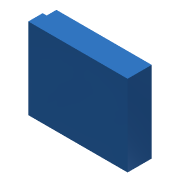
# Autodesk Inventor part: body_encoder
Saved by Autodesk Inventor 2014 (Build 180170000, 170)
## iProperties
Created: 2015-11-19
Part Number: body_encoder
Material: Generic
Document SubType Name: Modeling
Designer: Tom
Density: 1 g/cm^3
Appearance: Default
Author: Tom
Autodesk Inventor part; units mm, degrees
ref_plane "YZ Plane" through (0, 0, 0) normal (1, 0, 0) x (0, 1, 0)
ref_plane "XZ Plane" through (0, 0, 0) normal (0, 1, 0) x (-1, 0, 0)
sketch "Sketch1" plane through (0, 0, 0) normal (0, 0, 1) x (1, 0, 0)
  line L0 (0, 0) -> (12.6492, 0)
  line L1 (12.6492, 0) -> (12.6492, 11.176)
  line L2 (12.6492, 11.176) -> (0, 11.176)
  line L3 (0, 11.176) -> (0, 0)
  dimension "d0" = 12.6492
  dimension "d1" = 11.176
  constraints: 8 end point, 2 parallel, 1 horizontal, 1 perpendicular
  measures "d0" distance of L2.end L1.end
  measures "d1" distance of L1.end L0.end
extrude "Extrusion1" add sketch "Sketch1" along normal blind 3.9624
sketch "Sketch2" plane through (0, 0, 0) normal (-1, 0, 0) x (0, 0, 1)
  line L0 (0, 0) -> (3.9624, 0) projected
  line L1 (3.9624, 11.176) -> (2.0574, 11.176)
  line L2 (2.0574, 11.176) -> (2.0574, 0)
  line L3 (2.0574, 0) -> (3.9624, 0)
  line L4 (3.9624, 0) -> (3.9624, 11.176)
  dimension "d4" = 1.905
  constraints: 8 end point, 2 parallel, 1 horizontal, 1 perpendicular, 1 point on line
  measures "d4" distance of L3.end L2.end
ref_plane "Work Plane1" through (-0.5334, -0.3048, 5.08) normal (-1, 0, 0) x (0, 0, 1)
extrude "Extrusion2" add sketch "Sketch2" along normal up to surface (0.5334 mm away)
move faces "Move Face1" translate (0, 0.4064, 0) faces at (8.4328, 0, 2.0066)
move faces "Move Face2" translate (0, 0, 0.762) faces at (4.2164, 7.5861, 0)
body "Solid1"
